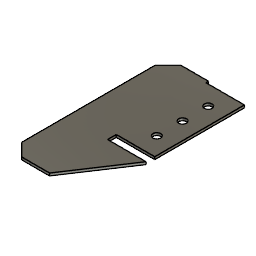
GPL H400 to H250G38 (Autodesk Fusion 360 design; units mm, degrees)
Autodesk Fusion 360 part; units mm, degrees
sketch "スケッチ1" plane through (0, 0, 0) normal (0, 0, 1) x (1, 0, 0)
  line L0 (2.5, 186) -> (-92.5, 186)
  line L1 (-92.5, 186) -> (-92.5, -186)
  line L2 (-92.5, -186) -> (2.5, -186)
  line L3 (92.5, -30) -> (92.5, 180)
  line L4 (89.5161, 180) -> (-92.5, -186) construction
  line L5 (-92.5, 186) -> (53.8847, -108.352) construction
  line L6 (2.5, 186) -> (2.5, 180)
  line L7 (2.5, 180) -> (92.5, 180)
  line L8 (-92.5, -186) -> (2.5, -186) construction
  line L9 (92.5, -50) -> (2.5, -186)
  line L10 (92.5, -50) -> (2.5, -50)
  line L11 (2.5, -50) -> (2.5, -30)
  line L12 (2.5, -30) -> (92.5, -30)
  dimension "d2" = 372
  dimension "d5" = 95
  dimension "d7" = 90
  dimension "d8" = 20
  constraint horizontal L0
  constraint perpendicular L0 L1
  constraint parallel L0 L2
  constraint parallel L1 L3
  constraint coincident L4 origin
  constraint coincident L5 origin
  constraint vertical L6
  constraint horizontal L7
  constraint coincident L7 L4.start
  constraint perpendicular L1 L8
  constraint coincident L9 L5.end
  constraint horizontal L10
  constraint vertical L11
  constraint horizontal L12
  measures "d2" distance of L0.end L1.end
  measures "d5" distance of L1.end L2.end
  measures "d7" distance of L9.start L10.end
  measures "d8" distance of L9.start L3.start
extrude "押し出し1" add sketch "スケッチ1" along normal blind 6
chamfer "面取り1" distance 30 angle 45 2 edges at (-92.5, -186, 3) (-92.5, 186, 3)
sketch "スケッチ2" plane through (0, 0, 6) normal (0, 0, 1) x (-1, 0, 0)
  line L0 (62.5, -186) -> (92.5, -156)
  line L1 (92.5, -156) -> (92.5, 156)
  line L2 (92.5, 156) -> (62.5, 186)
  line L3 (62.5, 186) -> (-2.5, 186)
  line L4 (-2.5, 186) -> (-92.5, 50)
  line L5 (-92.5, 50) -> (-2.5, 50)
  line L6 (-2.5, 50) -> (-2.5, 30)
  line L7 (-2.5, 30) -> (-92.5, 30)
  line L8 (-92.5, 30) -> (-92.5, -180)
  line L9 (-92.5, -180) -> (-2.5, -180)
  line L10 (-2.5, -180) -> (-2.5, -186)
  line L11 (-2.5, -186) -> (62.5, -186)
  line L12 (-92.5, -180) -> (-52.5, -180) construction
  line L13 (-52.5, -180) -> (-52.5, -135) construction
  line L14 (-52.5, -135) -> (-92.5, -135) construction
  line L15 (-92.5, -135) -> (-92.5, -180) construction
  line L16 (-52.5, -135) -> (-52.5, -75) construction
  line L17 (-52.5, -75) -> (-52.5, -15) construction
  point P0 (-52.5, -135)
  point P1 (-52.5, -75)
  dimension "d12" = 40
  dimension "d13" = 45
  dimension "d14" = 60
  dimension "d15" = 60
  constraint horizontal L12
  constraint vertical L13
  constraint horizontal L14
  constraint vertical L15
  constraint coincident L8.end L9.start
  constraint perpendicular L14 L16
  constraint parallel L16 L17
  constraint coincident P0 L13.end
  constraint coincident P1 L16.end
  measures "d12" distance of L8.end L12.end
  measures "d13" distance of L8.end L14.end
  measures "d14" distance of P0 P1
  measures "d15" distance of P1 L17.end
hole "穴1" at (52.5, 135, 6) at (52.5, 75, 6) at (52.5, 15, 6) direction (0, 0, -1) diameter 18 end through all
equation "d5 = 30 mm + 65 mm"
